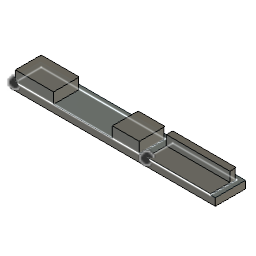
co2_o2_insert (Autodesk Fusion 360 design; units mm, degrees)
part number: 2026-03-23-11-19-43-358
Autodesk Fusion 360 part; units mm, degrees
sketch "Sketch1" plane through (0, 0, 0) normal (0, 0, 1) x (1, 0, 0)
  line L0 (0, 0) -> (95, 0)
  line L1 (95, 0) -> (95, 14)
  line L2 (95, 14) -> (0, 14)
  line L3 (0, 14) -> (0, 0)
  dimension "d1" = 95
  dimension "d2" = 14
  constraint horizontal L0
  constraint vertical L1
  constraint horizontal L2
  constraint vertical L3
  constraint coincident L0.start L3.end
  measures "d1" distance of L0.start L0.end
  measures "d2" distance of L0.start L2.end
extrude "Extrude1" add sketch "Sketch1" along normal blind 3.5
sketch "Sketch2" plane through (0, 0, 3.5) normal (0, 0, 1) x (-1, 0, 0)
  line L0 (0, -14) -> (0, 0)
  line L1 (0, 0) -> (-95, 0)
  line L2 (-95, 0) -> (-95, -14)
  line L3 (-95, -14) -> (0, -14)
  line L4 (-2.25, 0) -> (-59.75, 0)
  line L5 (-59.75, 0) -> (-59.75, -12)
  line L6 (-59.75, -12) -> (-2.25, -12)
  line L7 (-2.25, -12) -> (-2.25, 0)
  line L8 (-63.25, 0) -> (-92.75, 0)
  line L9 (-92.75, 0) -> (-92.75, -12)
  line L10 (-92.75, -12) -> (-63.25, -12)
  line L11 (-63.25, -12) -> (-63.25, 0)
  dimension "d5" = 57.5
  dimension "d6" = 12
  dimension "d7" = 2.25
  dimension "d8" = 29.5
  dimension "d9" = 12
  dimension "d22" = 2.25
  constraint horizontal L4
  constraint vertical L5
  constraint horizontal L6
  constraint vertical L7
  constraint coincident L1 L4.start
  constraint horizontal L8
  constraint vertical L9
  constraint horizontal L10
  constraint vertical L11
  constraint coincident L1 L8.start
  measures "d5" distance of L4.start L4.end
  measures "d6" distance of L4.start L6.end
  measures "d7" distance of L0 L7
  measures "d8" distance of L8.start L8.end
  measures "d9" distance of L8.start L10.end
  measures "d22" distance of L2 L9
extrude "Extrude6" add sketch "Sketch2" along normal blind 0.5 contours L1 L8 L9 L10 L11
extrude "Extrude7" add sketch "Sketch2" along normal blind 5 contours L1 L4 L5 L6 L7
sketch "Sketch5" plane through (0, 0, 4) normal (0, 0, 1) x (-1, 0, 0)
  line L0 (-63.25, -12) -> (-63.25, 0)
  line L1 (-63.25, 0) -> (-92.75, 0)
  line L2 (-92.75, 0) -> (-92.75, -12)
  line L3 (-92.75, -12) -> (-63.25, -12)
  line L4 (-63.25, -12) -> (-92.75, -12)
  line L5 (-92.75, -12) -> (-92.75, -9)
  line L6 (-92.75, -9) -> (-63.25, -9)
  line L7 (-63.25, -9) -> (-63.25, -12)
  dimension "d27" = 3
  constraint horizontal L4
  constraint vertical L5
  constraint horizontal L6
  constraint vertical L7
  constraint coincident L0.start L3.end
  measures "d27" distance of L0.start L6.end
extrude "Extrude8" add sketch "Sketch5" along normal blind 4.5 contours L0 L2 L3 L4 L5 L6 L7
sketch "Sketch6" plane through (0, 0, 8.5) normal (0, 0, 1) x (-1, 0, 0)
  line L0 (-2.25, -12) -> (-2.25, 0)
  line L1 (-2.25, 0) -> (-59.75, 0)
  line L2 (-59.75, 0) -> (-59.75, -12)
  line L3 (-59.75, -12) -> (-2.25, -12)
  line L4 (-20, -12) -> (-47.25, -12)
  line L5 (-47.25, -12) -> (-47.25, 0)
  line L6 (-47.25, 0) -> (-20, 0)
  line L7 (-20, 0) -> (-20, -12)
  line L8 (-2.25, -12) -> (-2.25, 0)
  dimension "d30" = 17.75
  dimension "d31" = 27.25
  constraint horizontal L4
  constraint vertical L5
  constraint horizontal L6
  constraint vertical L7
  constraint coincident L1 L5.end
  constraint coincident L3 L4.start
  measures "d30" distance of L7 L8
  measures "d31" distance of L4.start L4.end
extrude "Extrude9" cut sketch "Sketch6" against normal blind 5 contours L1 L3 L4 L5 L6 L7
fillet "Fillet1" radius 0.5 6 edges at (92.75, 12, 6) (63.25, 12, 6) (47.25, 12, 6) (20, 12, 6) (2.25, 12, 6) (59.75, 12, 6)
